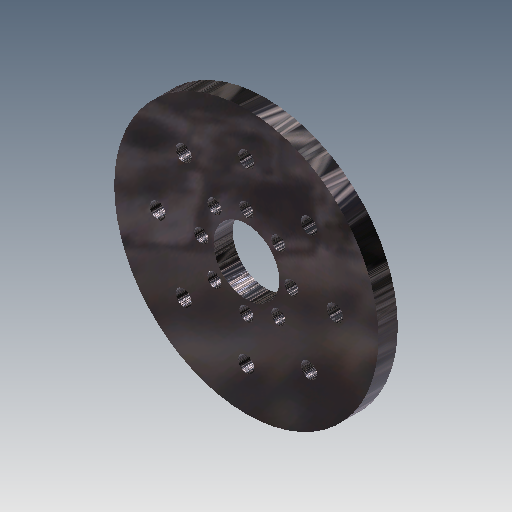
# Autodesk Inventor part: 出力部品A_ダブルスラスト用(t2_アルミ)
Saved by Autodesk Inventor 2019.4 (Build 234330000, 330)
## iProperties
Created: 2018-08-09
Part Number: 出力部品A_ダブルスラスト用(t2_アルミ)
Material: アルミニウム 6061
Document SubType Name: Modeling
Designer: Owner
Density: 2.7 g/cm^3
Appearance: アルミニウム - フラット
Mass: 9.46777 g
Surface Area: 31.7464 cm^2
Volume: 3.50658 cm^3
Author: Owner
Autodesk Inventor part; units mm, degrees
ref_plane "YZ Plane" through (0, 0, 0) normal (1, 0, 0) x (0, 1, 0)
ref_plane "XZ Plane" through (0, 0, 0) normal (0, 1, 0) x (-1, 0, 0)
ref_plane "XY Plane" through (0, 0, 0) normal (0, 0, 1) x (1, 0, 0)
sketch "スケッチ1" plane through (0, 0, 0) normal (0, 0, 1) x (1, 0, 0)
  circle A0 centre (0, 0) radius 20.5
  circle A1 centre (0, 0) radius 10 construction
  circle A2 centre (0, 0) radius 7 construction
  circle A3 centre (0, -7) radius 1.1
  circle A4 centre (4.9497, -4.9497) radius 1.1
  circle A5 centre (7, 0) radius 1.1
  circle A6 centre (4.9497, 4.9497) radius 1.1
  circle A7 centre (0, 7) radius 1.1
  circle A8 centre (-4.9497, 4.9497) radius 1.1
  circle A9 centre (-7, 0) radius 1.1
  circle A10 centre (-4.9497, -4.9497) radius 1.1
  circle A11 centre (0, 0) radius 15.5 construction
  circle A12 centre (0, 0) radius 12 construction
  line L0 (0, -12) -> (0, -15.5) construction
  circle A13 centre (0, -13.75) radius 1.25
  circle A14 centre (43.1211, 8.0958) radius 5 projected
  circle A15 centre (46.9662, 2.2465) radius 0.8 projected
  circle A16 centre (49.9761, 6.6786) radius 0.8 projected
  circle A17 centre (48.9705, 11.9409) radius 0.8 projected
  circle A18 centre (44.5383, 14.9509) radius 0.8 projected
  circle A19 centre (39.276, 13.9452) radius 0.8 projected
  circle A20 centre (36.2661, 9.513) radius 0.8 projected
  circle A21 centre (37.2717, 4.2507) radius 0.8 projected
  circle A22 centre (41.7039, 1.2408) radius 0.8 projected
  circle A23 centre (43.1211, 8.0958) radius 10 projected
  circle A24 centre (0, 0) radius 5.1
  circle A25 centre (0, 0) radius 13.75 construction
  circle A26 centre (9.7227, -9.7227) radius 1.25
  circle A27 centre (13.75, 0) radius 1.25
  circle A28 centre (9.7227, 9.7227) radius 1.25
  circle A29 centre (0, 13.75) radius 1.25
  circle A30 centre (-9.7227, 9.7227) radius 1.25
  circle A31 centre (-13.75, 0) radius 1.25
  circle A32 centre (-9.7227, -9.7227) radius 1.25
  dimension "d2" = 14
  dimension "d6" = 360
  dimension "d0" = 41
  dimension "d1" = 20
  dimension "d3" = 2.2
  dimension "d8" = 5
  dimension "d10" = 2.5
  dimension "d15" = 10.2
  dimension "d18" = 27.5
  dimension "d19" = 13.75
  dimension "d22" = 360
  constraints: 20 centre point, 5 coincident, 3 vertical alignment, 2 end point, 1 midpoint, 1 vertical, 40 other
  measures "d0" diameter of A0
  measures "d1" diameter of A1
  measures "d3" diameter of A3
  measures "d10" diameter of A13
  measures "d15" diameter of A24
  measures "d18" diameter of A25
  measures "d19" distance of point (0, 0) A13.centre
extrude "押し出し2" add sketch "スケッチ1" along normal blind 3 contours A0
